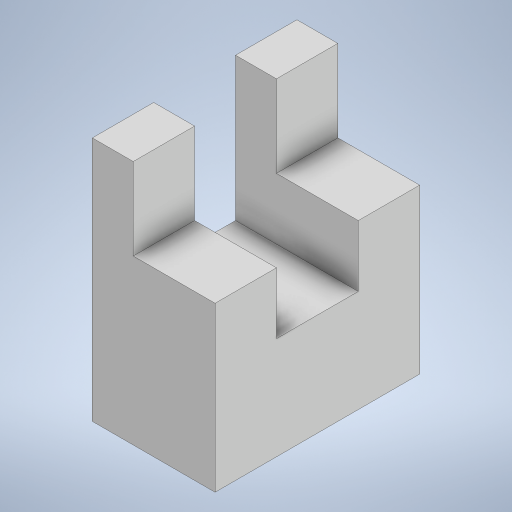
# Autodesk Inventor part: BT006_Prisma01
Saved by Autodesk Inventor 2023 (Build 270158000, 158)
## iProperties
Created: 2022-04-26
Part Number: BT006_Prisma01
Material: Generic
Document SubType Name: Modeling
Designer: Altar
Density: 1 g/cm^3
Appearance: Default
Author: Altar
Autodesk Inventor part; units mm, degrees
ref_plane "YZ Plane" through (0, 0, 0) normal (1, 0, 0) x (0, 1, 0)
ref_plane "XZ Plane" through (0, 0, 0) normal (0, 1, 0) x (-1, 0, 0)
ref_plane "XY Plane" through (0, 0, 0) normal (0, 0, 1) x (1, 0, 0)
sketch "Sketch1" plane through (0, 0, 0) normal (1, 0, 0) x (0, 1, 0)
  line L0 (-20.0775, -33.0426) -> (39.9225, -33.0426)
  line L1 (39.9225, -33.0426) -> (39.9225, -18.0426)
  line L2 (39.9225, -18.0426) -> (4.9225, -18.0426)
  line L3 (4.9225, -18.0426) -> (4.9225, 1.9574)
  line L4 (4.9225, 1.9574) -> (39.9225, 1.9574)
  line L5 (39.9225, 1.9574) -> (39.9225, 16.9574)
  line L6 (39.9225, 16.9574) -> (-20.0775, 16.9574)
  line L7 (-20.0775, 16.9574) -> (-20.0775, -33.0426)
  point P0 (0, 0)
  dimension "d0" = 50
  dimension "d1" = 15
  dimension "d2" = 15
  dimension "d3" = 25
  dimension "d4" = 60
  constraints: 16 end point, 6 perpendicular, 2 point on line, 1 horizontal
  measures "d0" distance of L6.end L0.start
  measures "d1" distance of L4.end L5.end
  measures "d2" distance of L0.end L1.end
  measures "d3" distance between parallel lines of L7 L3
  measures "d4" distance of L0.start L0.end
extrude "Extrusion1" add sketch "Sketch1" along normal blind 30
sketch "Sketch2" plane through (0, -20.0775, 16.9574) normal (0, 0, 1) x (1, 0, 0)
  line L0 (0, 60) -> (30, 60) projected
  line L1 (10, 60) -> (10, 40)
  line L2 (10, 40) -> (30, 40)
  line L3 (30, 60) -> (30, 0) projected
  line L4 (30, 60) -> (10, 60)
  point P0 (0, 20.0775)
  dimension "d7" = 20
  dimension "d8" = 20
  constraints: 6 end point, 2 point on line, 1 parallel, 1 perpendicular, 1 vertical
  measures "d7" distance of L1.end L2.end
  measures "d8" distance of L1.start L1.end
extrude "Extrusion2" cut sketch "Sketch2" against normal blind 60
body "Solid1"
